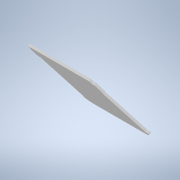
# Autodesk Inventor part: Rampa
Saved by Autodesk Inventor 2020.1 (Build 241239000, 239)
## iProperties
Created: 2019-12-08
Part Number: Rampa
Material: Generic
Document SubType Name: Modeling
Designer: Daniel
Density: 1 g/cm^3
Appearance: Default
Author: Daniel
Autodesk Inventor part; units mm, degrees
ref_plane "YZ Plane" through (0, 0, 0) normal (1, 0, 0) x (0, 1, 0)
ref_plane "XZ Plane" through (0, 0, 0) normal (0, 1, 0) x (-1, 0, 0)
ref_plane "XY Plane" through (0, 0, 0) normal (0, 0, 1) x (1, 0, 0)
sketch "Sketch2" plane through (0, 0, 0) normal (1, 0, 0) x (0, 1, 0)
  line L0 (-35, 40) -> (-35, -40)
  line L1 (-35, -40) -> (35, -40)
  line L2 (35, -40) -> (35, 40)
  line L3 (-65, -89.1286) -> (-63.153, -91.4926)
  line L4 (-63.153, -91.4926) -> (35, -14.8071)
  line L5 (-65, -89.1286) -> (-65, -32.0227)
  line L6 (-65, -32.0227) -> (-35, -8.5842)
  circle A0 centre (0, 5) radius 17.5
  circle A1 centre (0, 5) radius 31
  line L7 (-65, -89.1286) -> (35, -11)
  line L8 (29.4839, -19.1167) -> (27.6369, -16.7527)
  line L9 (12.9357, -32.0456) -> (11.0887, -29.6815)
  line L10 (0, 86.854) -> (0, -115.2189) construction
  line L11 (-162.2306, 0) -> (125.0958, 0) construction
  line L12 (34.212, -15.4227) -> (32.365, -13.0587)
  point P0 (0, 0)
  dimension "d0" = 38
  dimension "d2" = 80
  dimension "d3" = 29
  dimension "d7" = 70
  dimension "d8" = 30
  dimension "d9" = 35
  dimension "d10" = 62
  dimension "d11" = 35
  dimension "d12" = 35
  dimension "d15" = 5
  dimension "d16" = 3
  dimension "d17" = 21
  dimension "d18" = 7
  dimension "d19" = 45
  dimension "d24" = 86.854
  dimension "d25" = 115.219
  dimension "d26" = 6
  constraints: 26 end point, 8 point on line, 6 parallel, 4 perpendicular, 3 vertical, 2 centre point, 2 horizontal, 2 other
  measures "d0" angle of L1 L4
  measures "d2" distance from line of L2.end L1
  measures "d3" distance from line of L7.end L1
  measures "d7" distance between parallel lines of L0 L2
  measures "d8" distance between parallel lines of L0 L5
  measures "d9" diameter of A0
  measures "d10" diameter of A1
  measures "d11" distance from line of L2 A0.centre
  measures "d12" horizontal distance of L0.start A0.centre
  measures "d15" distance from line of L11 A0.centre
  measures "d16" distance between parallel lines of L4 L7
  measures "d17" distance between parallel lines of L9 L8
  measures "d18" distance from line of L4.end L8
  measures "d19" distance between parallel lines of L7 L6
  measures "d24" distance from line of L10.start L11
  measures "d25" distance from line of L10.end L11
  measures "d26" distance between parallel lines of L8 L12
extrude "Extrusion1" add sketch "Sketch2" along normal blind 82 contours L7 L9 L4 L1 | L1 L4 L3 L7 | L7 L8 L4 L9 | L7 L12 L4 L8
extrude "Extrusion2" add sketch "Sketch2" against normal blind 3 contours L7 L8 L4 L9
ref_plane "Work Plane1" through (41, 0, 0) normal (-1, 0, 0) x (0, 0, 1)
mirror "Mirror1" about plane through (41, 0, 0) normal (-1, 0, 0) of "Extrusion2"
sketch "Sketch3" plane through (82, 34.212, -15.4227) normal (0, 0.6156615, -0.7880108) x (-1, 0, 0)
  line L0 (82, -123.558) -> (0, -123.558) projected
  line L1 (-3, -123.558) -> (85, -123.558)
  line L2 (82, -123.558) -> (82, -27) projected
  line L3 (0, -123.558) -> (0, -27) projected
  line L4 (-3, -133.558) -> (85, -133.558)
  line L5 (-3, -123.558) -> (-3, -133.558)
  line L6 (85, -123.558) -> (85, -133.558)
  point P0 (82, -17.4642)
  point P1 (82, -123.558)
  point P2 (0, -123.558)
  dimension "d31" = 3
  dimension "d32" = 3
  dimension "d33" = 10
  constraints: 8 end point, 2 parallel, 1 collinear, 1 horizontal, 1 vertical
  measures "d31" distance from line of L2 L1.end
  measures "d32" distance from line of L3 L1.start
  measures "d33" distance between parallel lines of L1 L4
extrude "Extrusion3" add sketch "Sketch3" against normal up to surface (3 mm away)
fillet "Fillet1" radius 10 2 edges at (85, -71.9566, -96.4672) (-3, -71.9566, -96.4672)
body "Solid1"
